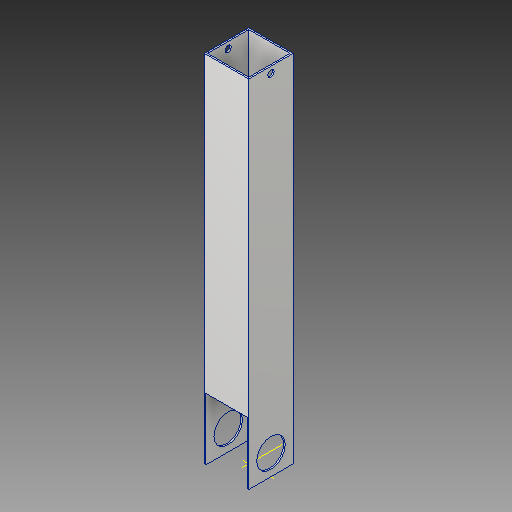
# Autodesk Inventor part: CAR_025_KickerBar
Saved by Autodesk Inventor 2018.3 (Build 223284000, 284)
## iProperties
Created: 2020-02-03
Part Number: CAR_025_KickerBar
Material: Aluminum 6061
Document SubType Name: Modeling
Designer: user
Mass: 234.084 g
Surface Area: 1105.11 cm^2
Volume: 86.6978 cm^3
Density: 2.7 g/cm^3
Appearance: Aluminum - Flat
Author: user
Autodesk Inventor part; units mm, degrees
ref_plane "YZ Plane" through (0, 0, 0) normal (1, 0, 0) x (0, 1, 0)
ref_plane "XZ Plane" through (0, 0, 0) normal (0, 1, 0) x (-1, 0, 0)
ref_plane "XY Plane" through (0, 0, 0) normal (0, 0, 1) x (1, 0, 0)
sketch "Sketch1" plane through (0, 0, 0) normal (0, 1, 0) x (-1, 0, 0)
  line L0 (0, 0) -> (44.45, 0)
  line L1 (44.45, 0) -> (44.45, -44.45)
  line L2 (44.45, -44.45) -> (0, -44.45)
  line L3 (0, -44.45) -> (0, 0)
  line L4 (42.8625, -1.5875) -> (1.5875, -1.5875)
  line L5 (1.5875, -1.5875) -> (1.5875, -42.8625)
  line L6 (1.5875, -42.8625) -> (42.8625, -42.8625)
  line L7 (42.8625, -42.8625) -> (42.8625, -1.5875)
  dimension "d0" = 44.45
  dimension "d2" = 1.5875
  constraints: 16 end point, 4 parallel, 3 perpendicular, 1 horizontal, 3 other
  measures "d0" distance of L1.end L2.end
  measures "d2" distance between parallel lines of L0 L4
extrude "Extrusion1" add sketch "Sketch1" along normal mid plane 356.1949
ref_plane "Work Plane1" through (-22.225, -178.0974, -44.45) normal (1, 0, 0) x (0, 0, -1)
sketch "Sketch2" plane through (-44.45, -178.0974, 0) normal (-1, 0, 0) x (0, 0, 1)
  line L0 (-44.45, 356.1949) -> (0, 356.1949) projected
  line L1 (0, 356.1949) -> (0, 0) projected
  line L2 (-44.45, 356.1949) -> (-44.45, 0) projected
  point P0 (0, 178.0974)
  point P1 (-22.225, 349.8449)
  dimension "d5" = 6.35
  dimension "d17" = 22.225
  measures "d5" distance from line of L0 point (-22.225, 349.845)
  measures "d17" distance from line of L2 point (-22.225, 349.845)
hole "Hole1" at (-44.45, 171.7474, -22.225) direction (1, 0, 0) diameter 6.35 end through all
ref_plane "Work Plane2" through (-44.45, 178.0974, -22.225) normal (0, 0, 1) x (1, 0, 0)
sketch "Sketch3" plane through (-44.45, 178.0974, 0) normal (0, 0, 1) x (1, 0, 0)
  line L0 (44.45, -356.1949) -> (44.45, 0) projected
  line L1 (0, 0) -> (44.45, 0) projected
  line L2 (0, 0) -> (0, -356.1949) projected
  line L3 (44.45, -356.1949) -> (0, -356.1949) projected
  line L4 (1.5875, 0) -> (1.5875, -356.1949) projected
  line L5 (42.8625, -356.1949) -> (42.8625, 0) projected
  line L6 (1.5875, -356.1949) -> (42.8625, -356.1949) projected
  line L7 (1.5875, -356.1949) -> (42.8625, -356.1949)
  line L8 (42.8625, -356.1949) -> (42.8625, -294.2824)
  line L9 (42.8625, -294.2824) -> (1.5875, -294.2824)
  line L10 (1.5875, -294.2824) -> (1.5875, -356.1949)
  point P0 (44.45, -178.0974)
  dimension "d14" = 61.9125
  constraints: 8 end point, 2 parallel, 1 horizontal, 1 perpendicular, 1 point on line
  measures "d14" distance between parallel lines of L3 L9
extrude "Extrusion2" cut sketch "Sketch3" against normal through all contours L3 L4 L9 L5
sketch "Sketch4" plane through (-44.45, -178.0974, 0) normal (-1, 0, 0) x (0, 0, 1)
  line L0 (-44.45, 356.1949) -> (-44.45, 0) projected
  line L1 (0, 0) -> (-44.45, 0) projected
  point P0 (0, 178.0974)
  point P1 (-22.225, 20.6502)
  dimension "d18" = 22.225
  dimension "d19" = 20.6502
  measures "d18" distance from line of L0 point (-22.225, 20.65)
  measures "d19" distance from line of L1 point (-22.225, 20.65)
hole "Hole2" at (-44.45, -157.4472, -22.225) direction (1, 0, 0) diameter 28.575 end through all
body "Solid1"
